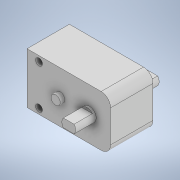
# Autodesk Inventor part: TT motor output
Saved by Autodesk Inventor 2022 (Build 260153070, 153G)
## iProperties
Created: 2021-11-27
Part Number: TT motor output
Material: Generic
Document SubType Name: Modeling
Designer: a laptop
Density: 1 g/cm^3
Appearance: Default
Author: a laptop
Autodesk Inventor part; units mm, degrees
ref_plane "YZ Plane" through (0, 0, 0) normal (1, 0, 0) x (0, 1, 0)
ref_plane "XZ Plane" through (0, 0, 0) normal (0, 1, 0) x (-1, 0, 0)
ref_plane "XY Plane" through (0, 0, 0) normal (0, 0, 1) x (1, 0, 0)
sketch "Sketch1" plane through (0, 0, 0) normal (0, 0, 1) x (1, 0, 0)
  line L0 (-14.5, 5.3996) -> (17.875, 5.3996)
  line L1 (22, 5.3996) -> (22, 1.2746)
  line L2 (22, -16.8504) -> (-14.5, -16.8504)
  line L3 (-14.5, -16.8504) -> (-14.5, -5.7254)
  line L4 (-14.5, -5.7254) -> (22, -5.7254) construction
  line L5 (-14.5, -5.7254) -> (-14.5, 5.3996)
  circle A0 centre (0, -5.7254) radius 2
  circle A1 centre (-9.25, 3.0246) radius 1.5
  arc A2 (22, 1.2746) -> (17.875, 5.3996) centre (17.875, 1.2746) ccw
  line L6 (17.875, 5.3996) -> (22, 5.3996)
  line L7 (22, 1.2746) -> (22, -16.8504)
  arc A3 (17.875, -16.8504) -> (22, -12.7254) centre (17.875, -12.7254) ccw
  circle A4 centre (-9.25, -14.4754) radius 1.5
  circle A5 centre (12.7, -5.7254) radius 2.9908
  line L8 (10.35, -3.8754) -> (15.05, -3.8754)
  line L9 (15.05, -7.5754) -> (10.35, -7.5754)
  point P0 (0, 0)
  dimension "d6" = 4
  dimension "d8" = 3
  dimension "d11" = 5.25
  dimension "d12" = 22.25
  dimension "d13" = 8.75
  dimension "d16" = 14.5
  dimension "d17" = 14
  dimension "d18" = 36.5
  dimension "d19" = 3.7
  constraints: 20 end point, 9 point on circle, 7 parallel, 6 centre point, 6 perpendicular, 6 point on line, 4 symmetric about line, 3 equal length, 3 horizontal, 2 tangent, 1 horizontal alignment, 1 vertical alignment, 2 other
  measures "d6" diameter of A0
  measures "d8" diameter of A1
  measures "d11" distance from line of L5 A1.centre
  measures "d12" distance of L1.start L2.start
  measures "d13" distance from line of L4 A1.centre
  measures "d16" distance from line of L3 A0.centre
  measures "d17" distance of A3.end A2.start
  measures "d18" distance of L0.start L1.start
  measures "d19" distance between parallel lines of L9 L8
extrude "Extrusion1" add sketch "Sketch1" along normal mid plane 18.5 contours L0 A2 L7 A3 L2 L3 L5
extrude "Extrusion2" add sketch "Sketch1" along normal mid plane 22.5 contours A0
extrude "Extrusion3" add sketch "Sketch1" along normal mid plane 20.5 contours A5 L9 L8 | L8 A5 | A5 L9
extrude "Extrusion4" add sketch "Sketch1" along normal mid plane 36.5 contours A5 L9 L8
sketch "Sketch2" plane through (-14.5, -16.8504, 9.25) normal (-1, 0, 0) x (0, 0, 1)
  point P0 (-9.25, 16.8504)
body "Solid1"
